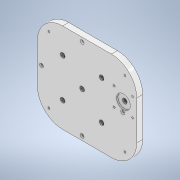
# Autodesk Inventor part: FourWireLitzBasePlate
Saved by Autodesk Inventor 2020.2 (Build 242310000, 310)
## iProperties
Created: 2020-03-15
Part Number: FourWireLitzBasePlate
Material: Generic
Document SubType Name: Modeling
Designer: elmar
Density: 1 g/cm^3
Appearance: White
Author: elmar
Autodesk Inventor part; units mm, degrees
ref_plane "YZ Plane" through (0, 0, 0) normal (1, 0, 0) x (0, 1, 0)
ref_plane "XZ Plane" through (0, 0, 0) normal (0, 1, 0) x (-1, 0, 0)
ref_plane "XY Plane" through (0, 0, 0) normal (0, 0, 1) x (1, 0, 0)
sketch "Sketch1" plane through (0, 0, 0) normal (0, 0, 1) x (1, 0, 0)
  line L0 (32.6, -32.6) -> (-32.6, -32.6)
  line L1 (-32.6, -32.6) -> (-32.6, 32.6)
  line L2 (-32.6, 32.6) -> (32.6, 32.6)
  line L3 (32.6, 32.6) -> (32.6, -32.6)
  line L4 (32.6, -32.6) -> (-32.6, 32.6) construction
  line L5 (-32.6, -32.6) -> (32.6, 32.6) construction
  line L6 (-67.9674, 0) -> (0, 67.9674)
  line L7 (0, 67.9674) -> (67.9674, 0)
  line L8 (67.9674, 0) -> (0, -67.9674)
  line L9 (0, -67.9674) -> (-67.9674, 0)
  line L10 (-108.2683, 0) -> (124.6095, 0) projected
  circle A0 centre (32.6, 32.6) radius 32.6
  circle A1 centre (69.1913, 15.9531) radius 7.6
  circle A2 centre (32.6, -32.6) radius 35
  circle A3 centre (69.1913, 15.9531) radius 10
  line L11 (53.6913, 31.4531) -> (84.6913, 31.4531)
  line L12 (84.6913, 31.4531) -> (84.6913, 0.4531)
  line L13 (84.6913, 0.4531) -> (53.6913, 0.4531)
  line L14 (53.6913, 0.4531) -> (53.6913, 31.4531)
  line L15 (90.3413, 37.1031) -> (90.3413, -5.1969)
  line L16 (90.3413, -5.1969) -> (48.0413, -5.1969)
  line L17 (48.0413, -5.1969) -> (48.0413, 37.1031)
  line L18 (48.0413, 37.1031) -> (90.3413, 37.1031)
  line L19 (-75, 75) -> (91.3413, 75)
  line L20 (91.3413, 75) -> (91.3413, -75)
  line L21 (91.3413, -75) -> (-75, -75)
  line L22 (-75, -75) -> (-75, 75)
  circle A4 centre (69.1913, 15.9531) radius 11.5
  circle A5 centre (67.9674, 0) radius 6
  point P0 (0, 0)
  point P1 (0, 0)
  point P2 (-75, 0)
  dimension "d0" = 65.2
  dimension "d1" = 67.9674
  dimension "d2" = 65.2
  dimension "d3" = 15.2
  dimension "d4" = 70
  dimension "d5" = 20
  dimension "d7" = 31
  dimension "d8" = 42.3
  dimension "d9" = 150
  dimension "d10" = 1
  dimension "d11" = 7.0326
  dimension "d12" = 7.0326
  dimension "d37" = 23
  dimension "d38" = 12
  dimension "d154" = 96.1204
  constraints: 44 end point, 8 coincident, 6 centre point, 4 parallel, 3 midpoint, 3 perpendicular, 2 horizontal, 2 point on line, 2 tangent, 2 vertical, 27 other
  measures "d0" distance of L1.end L2.end
  measures "d1" distance of point (0, 0) L6.start
  measures "d2" diameter of A0
  measures "d3" diameter of A1
  measures "d4" diameter of A2
  measures "d5" diameter of A3
  measures "d7" distance of L11.start L11.end
  measures "d8" distance of L17.end L15.start
  measures "d9" distance of L21.end L19.start
  measures "d10" distance between parallel lines of L20 L15
  measures "d11" distance from line of L19 L6.end
  measures "d12" distance from line of L22 L6.start
  measures "d37" diameter of A4
  measures "d38" diameter of A5
  measures "d154" distance of L8.end L6.start
extrude "Extrusion1" add sketch "Sketch1" along normal blind 10 contours L3 L10 A2 L17 L16 L8 L0 | L0 A2 L10 L3 | A2 L8 L9 L10 L1 L0 | L0 L1 L10 A2 | A0 A2 L3 | A0 A2 L10 | L10 A2 A0 | L3 A2 A0 | L10 L1 L2 A0 A2 | A2 L8 L16 A5 L15 L10 L20 L21 L22 L9 | L8 A2 | A2 A0 L2 L3 | L3 L2 A0 L7 L17 A2 | A2 A0 L17 L10 | L10 L17 A2 | L10 L6 L7 A0 L2 L1 | A2 L16 L8 | L17 A0 L14 L13 A5 L10 | L10 A5 L8 L16 A2 L17 | A2 L16 L17 | L17 L7 L14 A0 | L10 L22 L19 L20 L15 L18 A0 L7 L6 | L8 A5 L16 | A5 L13 L7 L10 | L10 L8 A5 | A0 L18 L17 L7 | L14 L7 A0 | A0 L7 A5 L13 L14 | L17 L18 A0 L11 L14 L7 | L8 L10 A5 L16 | L16 A5 | L7 L13 A5 L10 | A5 L7 L13 | L18 L15 L10 A5 L13 L12 L11 A0 | A0 A4 A5 L7 | L7 L14 L11 A0 A4 | A5 L10 L15 L16 | L7 A5 A4 L13 | A4 A0 A3 | A0 A3 A5 A4 | A5 A4 A0 L11 L12 L13 | A5 A4 | A3 A0 | A1 | A0 A3 | A4 A5 A3 A0
fillet "Fillet1" radius 42.4 4 edges at (-75, 75, 5) (91.3413, 75, 5) (91.3413, -75, 5) (-75, -75, 5)
hole "Hole1" at (84.6913, 31.4531, 0) at (53.6913, 31.4531, 0) at (53.6913, 0.4531, 0) at (84.6913, 0.4531, 0) direction (0, 0, 1) diameter 3.2 depth 10 tip angle 118 countersink diameter 6.5 countersink angle 90 clearance for "Flat Head Machine Screw" size "M3" standard "Ansi Metric M Profile"
sketch "Sketch2" plane through (0, 0, 10) normal (0, 0, 1) x (1, 0, 0)
  circle A0 centre (69.1913, 15.9531) radius 11.5 projected
  point P0 (0, 0)
  point P1 (0, 67.9674)
  point P2 (-67.9674, 0)
  point P3 (0, -67.9674)
  point P4 (67.9674, 0)
hole "Hole2" at (0, 67.9674, 10) at (67.9674, 0, 10) at (0, -67.9674, 10) at (-67.9674, 0, 10) direction (0, 0, -1) diameter 3.2 depth 10 tip angle 118 countersink diameter 6.5 countersink angle 90 clearance for "Flat Head Machine Screw" size "M3" standard "Ansi Metric M Profile"
hole "Hole3" at (32.6, 32.6, 0) at (69.1913, 15.9531, 0) at (32.6, -32.6, 0) at (-32.6, -32.6, 0) at (-32.6, 32.6, 0) at (0, 0, 0) direction (0, 0, 1) diameter 8 depth 10 tip angle 118
extrude "Extrusion2" cut sketch "Sketch2" against normal blind 2.2
sketch "Sketch3" plane through (0, 0, 0) normal (0, 0, -1) x (-1, 0, 0)
  line L0 (-71.8515, 55.5103) -> (55.5103, 55.5103)
  line L1 (55.5103, 55.5103) -> (55.5103, -55.5103)
  line L2 (55.5103, -55.5103) -> (-71.8515, -55.5103)
  line L3 (-71.8515, -55.5103) -> (-71.8515, 55.5103)
  line L4 (-71.8515, 55.5103) -> (-78.9226, 62.5813)
  arc A0 (-48.9413, 75) -> (-91.3413, 32.6) centre (-48.9413, 32.6) ccw projected
  line L5 (120.5621, 0) -> (-136.9034, 0) projected
  line L6 (55.5103, 55.5103) -> (62.5813, 62.5813)
  arc A1 (75, 32.6) -> (32.6, 75) centre (32.6, 32.6) ccw projected
  circle A2 centre (-69.1913, 15.9531) radius 4 projected
  line L7 (-90.3413, 37.1031) -> (-48.0413, 37.1031)
  line L8 (-48.0413, 37.1031) -> (-48.0413, -5.1969)
  line L9 (-48.0413, -5.1969) -> (-90.3413, -5.1969)
  line L10 (-90.3413, -5.1969) -> (-90.3413, 37.1031)
  point P0 (0, 0)
  point P1 (-71.8515, 0)
  dimension "d41" = 135
  dimension "d42" = 10
  dimension "d50" = 42.3
  constraints: 20 end point, 3 perpendicular, 2 horizontal, 2 parallel, 2 point on circle, 2 point on line, 1 coincident, 1 midpoint, 9 other
  measures "d41" angle of L0 L4
  measures "d42" distance of L0.start L4.end
  measures "d50" distance of L9.end L7.start
hole "Hole4" at (71.8515, 55.5103, 0) at (-55.5103, 55.5103, 0) at (-55.5103, -55.5103, 0) at (71.8515, -55.5103, 0) direction (0, 0, 1) diameter 3.2 depth 10 tip angle 118 countersink diameter 6.5 countersink angle 90 clearance for "Flat Head Machine Screw" size "M3" standard "Ansi Metric M Profile"
sketch "Sketch12" plane through (0, 0, 0) normal (0, 0, -1) x (-1, 0, 0)
  line L0 (-52.2872, 53.0579) -> (-50, 53.0579) construction
  line L1 (-50, 53.0579) -> (-50, 50) construction
  line L2 (-50, 50) -> (-52.2872, 50) construction
  line L3 (-52.2872, 50) -> (-52.2872, 53.0579) construction
  line L4 (50, 53.1122) -> (52.2872, 53.1122) construction
  line L5 (52.2872, 53.1122) -> (52.2872, 50) construction
  line L6 (52.2872, 50) -> (50, 50) construction
  line L7 (50, 50) -> (50, 53.1122) construction
  line L8 (50, -50) -> (52.2872, -50) construction
  line L9 (52.2872, -50) -> (52.2872, -53.1764) construction
  line L10 (52.2872, -53.1764) -> (50, -53.1764) construction
  line L11 (50, -53.1764) -> (50, -50) construction
  line L12 (-52.2872, -50) -> (-50, -50) construction
  line L13 (-50, -50) -> (-50, -53.048) construction
  line L14 (-50, -53.048) -> (-52.2872, -53.048) construction
  line L15 (-52.2872, -53.048) -> (-52.2872, -50) construction
  line L16 (-50, 50) -> (50, 50)
  line L17 (50, 50) -> (50, -50)
  line L18 (50, -50) -> (-50, -50)
  line L19 (-50, -50) -> (-50, 50)
  spline S0 degree 2 poles (-51.2424, 52.7047) (-51.3536, 52.7047) (-51.5734, 52.6503) (-51.6796, 52.6083) knots 0 0 0 1 2 2 2
  spline S1 degree 2 poles (-51.6796, 52.6083) (-51.7784, 52.5663) (-51.9241, 52.4774) (-51.981, 52.4379) knots 0 0 0 1 2 2 2
  line L20 (-51.981, 52.4379) -> (-52.0057, 52.4379)
  line L21 (-52.0057, 52.4379) -> (-52.0057, 52.8702)
  spline S2 degree 2 poles (-52.0057, 52.8702) (-51.8723, 52.9418) (-51.4153, 53.0579) (-51.2103, 53.0579) knots 0 0 0 1 2 2 2
  spline S3 degree 2 poles (-51.2103, 53.0579) (-51.0028, 53.0579) (-50.6941, 52.9739) (-50.5681, 52.885) knots 0 0 0 1 2 2 2
  spline S4 degree 2 poles (-50.5681, 52.885) (-50.4347, 52.7886) (-50.2964, 52.5095) (-50.2964, 52.3218) knots 0 0 0 1 2 2 2
  spline S5 degree 2 poles (-50.2964, 52.3218) (-50.2964, 52.0699) (-50.6274, 51.6895) (-50.8596, 51.6401) knots 0 0 0 1 2 2 2
  line L22 (-50.8596, 51.6401) -> (-50.8596, 51.6105)
  spline S6 degree 2 poles (-50.8596, 51.6105) (-50.7632, 51.5907) (-50.5434, 51.5018) (-50.4495, 51.4128) knots 0 0 0 1 2 2 2
  spline S7 degree 2 poles (-50.4495, 51.4128) (-50.3557, 51.3264) (-50.2371, 51.0498) (-50.2371, 50.8497) knots 0 0 0 1 2 2 2
  spline S8 degree 2 poles (-50.2371, 50.8497) (-50.2371, 50.6447) (-50.3779, 50.2964) (-50.5064, 50.163) knots 0 0 0 1 2 2 2
  spline S9 degree 2 poles (-50.5064, 50.163) (-50.6397, 50.0247) (-51.0176, 49.8814) (-51.2572, 49.8814) knots 0 0 0 1 2 2 2
  spline S10 degree 2 poles (-51.2572, 49.8814) (-51.4869, 49.8814) (-51.9365, 49.9926) (-52.0896, 50.0692) knots 0 0 0 1 2 2 2
  line L23 (-52.0896, 50.0692) -> (-52.0896, 50.5014)
  line L24 (-52.0896, 50.5014) -> (-52.06, 50.5014)
  spline S11 degree 2 poles (-52.06, 50.5014) (-51.9316, 50.4076) (-51.4968, 50.2347) (-51.2819, 50.2347) knots 0 0 0 1 2 2 2
  spline S12 degree 2 poles (-51.2819, 50.2347) (-51.156, 50.2347) (-50.904, 50.3137) (-50.82, 50.4051) knots 0 0 0 1 2 2 2
  spline S13 degree 2 poles (-50.82, 50.4051) (-50.7385, 50.4965) (-50.6521, 50.7138) (-50.6521, 50.8793) knots 0 0 0 1 2 2 2
  spline S14 degree 2 poles (-50.6521, 50.8793) (-50.6521, 51.0448) (-50.7484, 51.2597) (-50.8349, 51.3215) knots 0 0 0 1 2 2 2
  spline S15 degree 2 poles (-50.8349, 51.3215) (-50.9213, 51.3832) (-51.156, 51.4301) (-51.2943, 51.4301) knots 0 0 0 1 2 2 2
  line L25 (-51.2943, 51.4301) -> (-51.4672, 51.4301)
  line L26 (-51.4672, 51.4301) -> (-51.4672, 51.7685)
  line L27 (-51.4672, 51.7685) -> (-51.3313, 51.7685)
  spline S16 degree 2 poles (-51.3313, 51.7685) (-51.0572, 51.7685) (-50.7114, 52.0304) (-50.7114, 52.2798) knots 0 0 0 1 2 2 2
  spline S17 degree 2 poles (-50.7114, 52.2798) (-50.7114, 52.3959) (-50.8003, 52.5614) (-50.8719, 52.6108) knots 0 0 0 1 2 2 2
  spline S18 degree 2 poles (-50.8719, 52.6108) (-50.9485, 52.6627) (-51.1362, 52.7047) (-51.2424, 52.7047) knots 0 0 0 1 2 2 2
  line L28 (52.1835, 51.1115) -> (51.8204, 51.1115)
  line L29 (51.8204, 51.1115) -> (51.8204, 50.0642)
  line L30 (51.8204, 50.0642) -> (51.4277, 50.0642)
  line L31 (51.4277, 50.0642) -> (51.4277, 51.1115)
  line L32 (51.4277, 51.1115) -> (50.0815, 51.1115)
  line L33 (50.0815, 51.1115) -> (50.0815, 51.5413)
  line L34 (50.0815, 51.5413) -> (51.445, 53.1122)
  line L35 (51.445, 53.1122) -> (51.8204, 53.1122)
  line L36 (51.8204, 53.1122) -> (51.8204, 51.44)
  line L37 (51.8204, 51.44) -> (52.1835, 51.44)
  line L38 (52.1835, 51.44) -> (52.1835, 51.1115)
  line L39 (51.4277, 51.44) -> (51.4277, 52.6306)
  line L40 (51.4277, 52.6306) -> (50.4026, 51.44)
  line L41 (50.4026, 51.44) -> (51.4277, 51.44)
  line L42 (-50.1853, -53.1122) -> (-52.0649, -53.1122)
  line L43 (-52.0649, -53.1122) -> (-52.0649, -52.68)
  spline S19 degree 2 poles (-52.0649, -52.68) (-51.8624, -52.4898) (-51.5018, -52.1366) (-51.3289, -51.9464) knots 0 0 0 1 2 2 2
  spline S20 degree 2 poles (-51.3289, -51.9464) (-50.9806, -51.5635) (-50.7262, -51.1041) (-50.7262, -50.8596) knots 0 0 0 1 2 2 2
  spline S21 degree 2 poles (-50.7262, -50.8596) (-50.7262, -50.7311) (-50.8052, -50.5385) (-50.8769, -50.4767) knots 0 0 0 1 2 2 2
  spline S22 degree 2 poles (-50.8769, -50.4767) (-50.9485, -50.415) (-51.1362, -50.3532) (-51.2498, -50.3532) knots 0 0 0 1 2 2 2
  spline S23 degree 2 poles (-51.2498, -50.3532) (-51.3585, -50.3532) (-51.5808, -50.4076) (-51.6821, -50.4495) knots 0 0 0 1 2 2 2
  spline S24 degree 2 poles (-51.6821, -50.4495) (-51.7685, -50.4841) (-51.9291, -50.5829) (-51.9785, -50.6175) knots 0 0 0 1 2 2 2
  line L44 (-51.9785, -50.6175) -> (-52.0007, -50.6175)
  line L45 (-52.0007, -50.6175) -> (-52.0007, -50.1828)
  spline S25 degree 2 poles (-52.0007, -50.1828) (-51.8747, -50.121) (-51.4227, -50) (-51.2202, -50) knots 0 0 0 1 2 2 2
  spline S26 degree 2 poles (-51.2202, -50) (-50.7929, -50) (-50.3112, -50.452) (-50.3112, -50.8373) knots 0 0 0 1 2 2 2
  spline S27 degree 2 poles (-50.3112, -50.8373) (-50.3112, -51.0176) (-50.3952, -51.319) (-50.4693, -51.4474) knots 0 0 0 1 2 2 2
  spline S28 degree 2 poles (-50.4693, -51.4474) (-50.5434, -51.5808) (-50.7583, -51.8426) (-50.8769, -51.9686) knots 0 0 0 1 2 2 2
  spline S29 degree 2 poles (-50.8769, -51.9686) (-51.0695, -52.1786) (-51.5413, -52.6281) (-51.6821, -52.759) knots 0 0 0 1 2 2 2
  line L46 (-51.6821, -52.759) -> (-50.1853, -52.759)
  line L47 (-50.1853, -52.759) -> (-50.1853, -53.1122)
  line L48 (51.9488, -53.0579) -> (50.4619, -53.0579)
  line L49 (50.4619, -53.0579) -> (50.4619, -52.7467)
  line L50 (50.4619, -52.7467) -> (51.0152, -52.7467)
  line L51 (51.0152, -52.7467) -> (51.0152, -50.704)
  line L52 (51.0152, -50.704) -> (50.4619, -50.704)
  line L53 (50.4619, -50.704) -> (50.4619, -50.4248)
  spline S30 degree 2 poles (50.4619, -50.4248) (50.7756, -50.4248) (51.072, -50.247) (51.0917, -50) knots 0 0 0 1 2 2 2
  line L54 (51.0917, -50) -> (51.4079, -50)
  line L55 (51.4079, -50) -> (51.4079, -52.7467)
  line L56 (51.4079, -52.7467) -> (51.9488, -52.7467)
  line L57 (51.9488, -52.7467) -> (51.9488, -53.0579)
  point P0 (0, 0)
  point P1 (0, 0)
  dimension "d131" = 100
  constraints: 8 end point, 5 coincident, 1 vertical, 17 other
  measures "d131" distance of L16.start L16.end
emboss "Emboss1" sketch "Sketch12" operation cut depth 0.3 direction (0, 0, 1) contours S0 S1 L20 L21 S2 S3 S4 S5 L22 S6 S7 S8 S9 S10 L23 L24 S11 S12 S13 S14 S15 L25 L26 L27 S16 S17 S18 | L28 L29 L30 L31 L32 L33 L34 L35 L36 L37 L38 | L42 L43 S19 S20 S21 S22 S23 S24 L44 L45 S25 S26 S27 S28 S29 L46 L47 | L48 L49 L50 L51 L52 L53 S30 L54 L55 L56 L57
thread "Thread6" size "M8x1.25" class "6H" standard "ANSI Metric M Profile" full length
thread "Thread7" size "M8x1.25" class "6H" standard "ANSI Metric M Profile" full length
thread "Thread8" size "M8x1.25" class "6H" standard "ANSI Metric M Profile" full length
thread "Thread9" size "M8x1.25" class "6H" standard "ANSI Metric M Profile" full length
thread "Thread10" size "M8x1.25" class "6H" standard "ANSI Metric M Profile" full length
sketch "Sketch48" plane through (32.6, 32.6, 10) normal (-1, 0, 0) x (0, 1, 0)
  line L0 (4, 0) -> (4, 10)
  line L1 (4, 10) -> (3.0732, 10)
  line L2 (3.0732, 10) -> (3.0732, 0)
  line L3 (3.0732, 0) -> (4, 0)
  line L4 (0, -2) -> (0, 12) projected
  constraints: 8 end point
revolve "Revolution21" add sketch "Sketch48" angle 360 about axis through (32.6, 32.6, 10) along (0, 0, -1) separate body
sketch "Sketch47" plane through (32.6, 36.6, 10) normal (1, 0, 0) x (0, 0, -1)
  line L0 (-0.7293, -0.0634) -> (-0.6251, -0.0634) construction
  line L1 (0.1041, -0.8638) -> (-0.0001, -1.0639) construction
  line L2 (-1.2501, -1.0639) -> (-1.3543, -0.8638) construction
  line L3 (-0.5209, -0.0634) -> (-0.6251, 0.1367) construction
  line L4 (-0.6251, 0.1367) -> (-0.7293, -0.0634) construction
  line L5 (-1.2501, -1.0639) -> (-1.1459, -0.8638) construction
  line L6 (-0.5209, -0.0634) -> (-0.1043, -0.8638)
  line L7 (-1.3543, -0.8638) -> (-1.1459, -0.8638) construction
  arc A0 (-1.3543, -0.8638) -> (-1.2501, -0.927) centre (-1.2501, -0.8096) ccw construction
  line L8 (0.1041, -0.8638) -> (-0.1043, -0.8638) construction
  line L9 (-1.2501, -1.0639) -> (-1.2501, -0.8638) construction
  line L10 (-0.0001, -1.0639) -> (-0.0001, -0.8638) construction
  line L11 (-0.6251, 0.1367) -> (-0.6251, -0.0002) construction
  line L12 (-1.2501, -0.927) -> (-0.0001, -0.927)
  arc A1 (-1.2501, -0.927) -> (-1.1459, -0.8638) centre (-1.2501, -0.8096) ccw
  line L13 (-0.1043, -0.8638) -> (-0.0001, -1.0639) construction
  line L14 (-1.1459, -0.8638) -> (-0.7293, -0.0634)
  line L15 (-0.0001, -0.0002) -> (-0.0001, 0.0177)
  line L16 (-0.0001, 0.0177) -> (-0.0001, -0.0002)
  line L17 (-0.0001, -0.0002) -> (0.0334, -0.0002)
  arc A2 (-0.1043, -0.8638) -> (-0.0001, -0.927) centre (-0.0001, -0.8096) ccw
  arc A3 (-0.0001, -0.927) -> (0.1041, -0.8638) centre (-0.0001, -0.8096) ccw construction
  arc A4 (-0.6251, -0.0002) -> (-0.7293, -0.0634) centre (-0.6251, -0.1176) ccw
  arc A5 (-0.5209, -0.0634) -> (-0.6251, -0.0002) centre (-0.6251, -0.1176) ccw
  line L18 (-0.6251, -0.0002) -> (-0.6251, -0.0634) construction
  line L19 (-0.6251, -0.0634) -> (-0.5209, -0.0634) construction
  dimension "d459" = 55
  dimension "d460" = 0.2001
  dimension "d461" = 0.2001
  dimension "Sketch47_ThreadOffset" = 0
  dimension "Sketch47_MajorRadius" = 0.9268
  dimension "d464" = 1.25
  dimension "Sketch47_MinorRadius" = 0
  constraints: 40 end point, 12 point on circle, 10 parallel, 8 tangent, 6 centre point, 6 collinear, 2 midpoint, 2 point on line, 1 horizontal, 1 perpendicular, 3 other
  measures "d459" angle of L6 L14
  measures "d460" distance of L3.end L0.end
  measures "d461" distance of L1.end L10.end
  measures "Sketch47_ThreadOffset" distance between parallel lines of L15 L10
  measures "Sketch47_MajorRadius" distance from line of L12 L15.start
  measures "d464" distance from line of L1.end L9
  measures "Sketch47_MinorRadius" distance edge to line of A5 L17
coil "Coil21" sketch "Sketch47" operation cut axis through (32.6, 32.6, 10) along (0, 0, -1) pitch 1.2513 turns 9.99001 hand right bodies 2
sketch "Sketch50" plane through (-32.6, 32.6, 10) normal (-1, 0, 0) x (0, 1, 0)
  line L0 (4, 0) -> (4, 10)
  line L1 (4, 10) -> (3.0732, 10)
  line L2 (3.0732, 10) -> (3.0732, 0)
  line L3 (3.0732, 0) -> (4, 0)
  line L4 (0, -2) -> (0, 12) projected
  constraints: 8 end point
revolve "Revolution22" add sketch "Sketch50" angle 360 about axis through (-32.6, 32.6, 10) along (0, 0, -1) separate body
sketch "Sketch49" plane through (-32.6, 36.6, 10) normal (1, 0, 0) x (0, 0, -1)
  line L0 (-0.7293, -0.0634) -> (-0.6251, -0.0634) construction
  line L1 (0.1041, -0.8638) -> (-0.0001, -1.0639) construction
  line L2 (-1.2501, -1.0639) -> (-1.3543, -0.8638) construction
  line L3 (-0.5209, -0.0634) -> (-0.6251, 0.1367) construction
  line L4 (-0.6251, 0.1367) -> (-0.7293, -0.0634) construction
  line L5 (-1.2501, -1.0639) -> (-1.1459, -0.8638) construction
  line L6 (-0.5209, -0.0634) -> (-0.1043, -0.8638)
  line L7 (-1.3543, -0.8638) -> (-1.1459, -0.8638) construction
  arc A0 (-1.3543, -0.8638) -> (-1.2501, -0.927) centre (-1.2501, -0.8096) ccw construction
  line L8 (0.1041, -0.8638) -> (-0.1043, -0.8638) construction
  line L9 (-1.2501, -1.0639) -> (-1.2501, -0.8638) construction
  line L10 (-0.0001, -1.0639) -> (-0.0001, -0.8638) construction
  line L11 (-0.6251, 0.1367) -> (-0.6251, -0.0002) construction
  line L12 (-1.2501, -0.927) -> (-0.0001, -0.927)
  arc A1 (-1.2501, -0.927) -> (-1.1459, -0.8638) centre (-1.2501, -0.8096) ccw
  line L13 (-0.1043, -0.8638) -> (-0.0001, -1.0639) construction
  line L14 (-1.1459, -0.8638) -> (-0.7293, -0.0634)
  line L15 (-0.0001, -0.0002) -> (-0.0001, 0.0177)
  line L16 (-0.0001, 0.0177) -> (-0.0001, -0.0002)
  line L17 (-0.0001, -0.0002) -> (0.0334, -0.0002)
  arc A2 (-0.1043, -0.8638) -> (-0.0001, -0.927) centre (-0.0001, -0.8096) ccw
  arc A3 (-0.0001, -0.927) -> (0.1041, -0.8638) centre (-0.0001, -0.8096) ccw construction
  arc A4 (-0.6251, -0.0002) -> (-0.7293, -0.0634) centre (-0.6251, -0.1176) ccw
  arc A5 (-0.5209, -0.0634) -> (-0.6251, -0.0002) centre (-0.6251, -0.1176) ccw
  line L18 (-0.6251, -0.0002) -> (-0.6251, -0.0634) construction
  line L19 (-0.6251, -0.0634) -> (-0.5209, -0.0634) construction
  dimension "d477" = 55
  dimension "d478" = 0.2001
  dimension "d479" = 0.2001
  dimension "Sketch49_ThreadOffset" = 0
  dimension "Sketch49_MajorRadius" = 0.9268
  dimension "d482" = 1.25
  dimension "Sketch49_MinorRadius" = 0
  constraints: 40 end point, 12 point on circle, 10 parallel, 8 tangent, 6 centre point, 6 collinear, 2 midpoint, 2 point on line, 1 horizontal, 1 perpendicular, 3 other
  measures "d477" angle of L6 L14
  measures "d478" distance of L3.end L0.end
  measures "d479" distance of L1.end L10.end
  measures "Sketch49_ThreadOffset" distance between parallel lines of L15 L10
  measures "Sketch49_MajorRadius" distance from line of L12 L15.start
  measures "d482" distance from line of L1.end L9
  measures "Sketch49_MinorRadius" distance edge to line of A5 L17
coil "Coil22" sketch "Sketch49" operation cut axis through (-32.6, 32.6, 10) along (0, 0, -1) pitch 1.2513 turns 9.99001 hand right bodies 3
sketch "Sketch52" plane through (0, 0, 10) normal (-1, 0, 0) x (0, 1, 0)
  line L0 (4, 0) -> (4, 10)
  line L1 (4, 10) -> (3.0732, 10)
  line L2 (3.0732, 10) -> (3.0732, 0)
  line L3 (3.0732, 0) -> (4, 0)
  line L4 (0, -2) -> (0, 12) projected
  constraints: 8 end point
revolve "Revolution23" add sketch "Sketch52" angle 360 about axis through (0, 0, 10) along (0, 0, -1) separate body
sketch "Sketch51" plane through (0, 4, 10) normal (1, 0, 0) x (0, 0, -1)
  line L0 (-0.7293, -0.0634) -> (-0.6251, -0.0634) construction
  line L1 (0.1041, -0.8638) -> (-0.0001, -1.0639) construction
  line L2 (-1.2501, -1.0639) -> (-1.3543, -0.8638) construction
  line L3 (-0.5209, -0.0634) -> (-0.6251, 0.1367) construction
  line L4 (-0.6251, 0.1367) -> (-0.7293, -0.0634) construction
  line L5 (-1.2501, -1.0639) -> (-1.1459, -0.8638) construction
  line L6 (-0.5209, -0.0634) -> (-0.1043, -0.8638)
  line L7 (-1.3543, -0.8638) -> (-1.1459, -0.8638) construction
  arc A0 (-1.3543, -0.8638) -> (-1.2501, -0.927) centre (-1.2501, -0.8096) ccw construction
  line L8 (0.1041, -0.8638) -> (-0.1043, -0.8638) construction
  line L9 (-1.2501, -1.0639) -> (-1.2501, -0.8638) construction
  line L10 (-0.0001, -1.0639) -> (-0.0001, -0.8638) construction
  line L11 (-0.6251, 0.1367) -> (-0.6251, -0.0002) construction
  line L12 (-1.2501, -0.927) -> (-0.0001, -0.927)
  arc A1 (-1.2501, -0.927) -> (-1.1459, -0.8638) centre (-1.2501, -0.8096) ccw
  line L13 (-0.1043, -0.8638) -> (-0.0001, -1.0639) construction
  line L14 (-1.1459, -0.8638) -> (-0.7293, -0.0634)
  line L15 (-0.0001, -0.0002) -> (-0.0001, 0.0177)
  line L16 (-0.0001, 0.0177) -> (-0.0001, -0.0002)
  line L17 (-0.0001, -0.0002) -> (0.0334, -0.0002)
  arc A2 (-0.1043, -0.8638) -> (-0.0001, -0.927) centre (-0.0001, -0.8096) ccw
  arc A3 (-0.0001, -0.927) -> (0.1041, -0.8638) centre (-0.0001, -0.8096) ccw construction
  arc A4 (-0.6251, -0.0002) -> (-0.7293, -0.0634) centre (-0.6251, -0.1176) ccw
  arc A5 (-0.5209, -0.0634) -> (-0.6251, -0.0002) centre (-0.6251, -0.1176) ccw
  line L18 (-0.6251, -0.0002) -> (-0.6251, -0.0634) construction
  line L19 (-0.6251, -0.0634) -> (-0.5209, -0.0634) construction
  dimension "d495" = 55
  dimension "d496" = 0.2001
  dimension "d497" = 0.2001
  dimension "Sketch51_ThreadOffset" = 0
  dimension "Sketch51_MajorRadius" = 0.9268
  dimension "d500" = 1.25
  dimension "Sketch51_MinorRadius" = 0
  constraints: 40 end point, 12 point on circle, 10 parallel, 8 tangent, 6 centre point, 6 collinear, 2 midpoint, 2 point on line, 1 horizontal, 1 perpendicular, 3 other
  measures "d495" angle of L6 L14
  measures "d496" distance of L3.end L0.end
  measures "d497" distance of L1.end L10.end
  measures "Sketch51_ThreadOffset" distance between parallel lines of L15 L10
  measures "Sketch51_MajorRadius" distance from line of L12 L15.start
  measures "d500" distance from line of L1.end L9
  measures "Sketch51_MinorRadius" distance edge to line of A5 L17
coil "Coil23" sketch "Sketch51" operation cut axis through (0, 0, 10) along (0, 0, -1) pitch 1.2513 turns 9.99001 hand right bodies 4
sketch "Sketch54" plane through (32.6, -32.6, 10) normal (-1, 0, 0) x (0, 1, 0)
  line L0 (4, 0) -> (4, 10)
  line L1 (4, 10) -> (3.0732, 10)
  line L2 (3.0732, 10) -> (3.0732, 0)
  line L3 (3.0732, 0) -> (4, 0)
  line L4 (0, -2) -> (0, 12) projected
  constraints: 8 end point
revolve "Revolution24" add sketch "Sketch54" angle 360 about axis through (32.6, -32.6, 10) along (0, 0, -1) separate body
sketch "Sketch53" plane through (32.6, -28.6, 10) normal (1, 0, 0) x (0, 0, -1)
  line L0 (-0.7293, -0.0634) -> (-0.6251, -0.0634) construction
  line L1 (0.1041, -0.8638) -> (-0.0001, -1.0639) construction
  line L2 (-1.2501, -1.0639) -> (-1.3543, -0.8638) construction
  line L3 (-0.5209, -0.0634) -> (-0.6251, 0.1367) construction
  line L4 (-0.6251, 0.1367) -> (-0.7293, -0.0634) construction
  line L5 (-1.2501, -1.0639) -> (-1.1459, -0.8638) construction
  line L6 (-0.5209, -0.0634) -> (-0.1043, -0.8638)
  line L7 (-1.3543, -0.8638) -> (-1.1459, -0.8638) construction
  arc A0 (-1.3543, -0.8638) -> (-1.2501, -0.927) centre (-1.2501, -0.8096) ccw construction
  line L8 (0.1041, -0.8638) -> (-0.1043, -0.8638) construction
  line L9 (-1.2501, -1.0639) -> (-1.2501, -0.8638) construction
  line L10 (-0.0001, -1.0639) -> (-0.0001, -0.8638) construction
  line L11 (-0.6251, 0.1367) -> (-0.6251, -0.0002) construction
  line L12 (-1.2501, -0.927) -> (-0.0001, -0.927)
  arc A1 (-1.2501, -0.927) -> (-1.1459, -0.8638) centre (-1.2501, -0.8096) ccw
  line L13 (-0.1043, -0.8638) -> (-0.0001, -1.0639) construction
  line L14 (-1.1459, -0.8638) -> (-0.7293, -0.0634)
  line L15 (-0.0001, -0.0002) -> (-0.0001, 0.0177)
  line L16 (-0.0001, 0.0177) -> (-0.0001, -0.0002)
  line L17 (-0.0001, -0.0002) -> (0.0334, -0.0002)
  arc A2 (-0.1043, -0.8638) -> (-0.0001, -0.927) centre (-0.0001, -0.8096) ccw
  arc A3 (-0.0001, -0.927) -> (0.1041, -0.8638) centre (-0.0001, -0.8096) ccw construction
  arc A4 (-0.6251, -0.0002) -> (-0.7293, -0.0634) centre (-0.6251, -0.1176) ccw
  arc A5 (-0.5209, -0.0634) -> (-0.6251, -0.0002) centre (-0.6251, -0.1176) ccw
  line L18 (-0.6251, -0.0002) -> (-0.6251, -0.0634) construction
  line L19 (-0.6251, -0.0634) -> (-0.5209, -0.0634) construction
  dimension "d513" = 55
  dimension "d514" = 0.2001
  dimension "d515" = 0.2001
  dimension "Sketch53_ThreadOffset" = 0
  dimension "Sketch53_MajorRadius" = 0.9268
  dimension "d518" = 1.25
  dimension "Sketch53_MinorRadius" = 0
  constraints: 40 end point, 12 point on circle, 10 parallel, 8 tangent, 6 centre point, 6 collinear, 2 midpoint, 2 point on line, 1 horizontal, 1 perpendicular, 3 other
  measures "d513" angle of L6 L14
  measures "d514" distance of L3.end L0.end
  measures "d515" distance of L1.end L10.end
  measures "Sketch53_ThreadOffset" distance between parallel lines of L15 L10
  measures "Sketch53_MajorRadius" distance from line of L12 L15.start
  measures "d518" distance from line of L1.end L9
  measures "Sketch53_MinorRadius" distance edge to line of A5 L17
coil "Coil24" sketch "Sketch53" operation cut axis through (32.6, -32.6, 10) along (0, 0, -1) pitch 1.2513 turns 9.99001 hand right bodies 5
sketch "Sketch56" plane through (-32.6, -32.6, 10) normal (-1, 0, 0) x (0, 1, 0)
  line L0 (4, 0) -> (4, 10)
  line L1 (4, 10) -> (3.0732, 10)
  line L2 (3.0732, 10) -> (3.0732, 0)
  line L3 (3.0732, 0) -> (4, 0)
  line L4 (0, -2) -> (0, 12) projected
  constraints: 8 end point
revolve "Revolution25" add sketch "Sketch56" angle 360 about axis through (-32.6, -32.6, 10) along (0, 0, -1) separate body
sketch "Sketch55" plane through (-32.6, -28.6, 10) normal (1, 0, 0) x (0, 0, -1)
  line L0 (-0.7293, -0.0634) -> (-0.6251, -0.0634) construction
  line L1 (0.1041, -0.8638) -> (-0.0001, -1.0639) construction
  line L2 (-1.2501, -1.0639) -> (-1.3543, -0.8638) construction
  line L3 (-0.5209, -0.0634) -> (-0.6251, 0.1367) construction
  line L4 (-0.6251, 0.1367) -> (-0.7293, -0.0634) construction
  line L5 (-1.2501, -1.0639) -> (-1.1459, -0.8638) construction
  line L6 (-0.5209, -0.0634) -> (-0.1043, -0.8638)
  line L7 (-1.3543, -0.8638) -> (-1.1459, -0.8638) construction
  arc A0 (-1.3543, -0.8638) -> (-1.2501, -0.927) centre (-1.2501, -0.8096) ccw construction
  line L8 (0.1041, -0.8638) -> (-0.1043, -0.8638) construction
  line L9 (-1.2501, -1.0639) -> (-1.2501, -0.8638) construction
  line L10 (-0.0001, -1.0639) -> (-0.0001, -0.8638) construction
  line L11 (-0.6251, 0.1367) -> (-0.6251, -0.0002) construction
  line L12 (-1.2501, -0.927) -> (-0.0001, -0.927)
  arc A1 (-1.2501, -0.927) -> (-1.1459, -0.8638) centre (-1.2501, -0.8096) ccw
  line L13 (-0.1043, -0.8638) -> (-0.0001, -1.0639) construction
  line L14 (-1.1459, -0.8638) -> (-0.7293, -0.0634)
  line L15 (-0.0001, -0.0002) -> (-0.0001, 0.0177)
  line L16 (-0.0001, 0.0177) -> (-0.0001, -0.0002)
  line L17 (-0.0001, -0.0002) -> (0.0334, -0.0002)
  arc A2 (-0.1043, -0.8638) -> (-0.0001, -0.927) centre (-0.0001, -0.8096) ccw
  arc A3 (-0.0001, -0.927) -> (0.1041, -0.8638) centre (-0.0001, -0.8096) ccw construction
  arc A4 (-0.6251, -0.0002) -> (-0.7293, -0.0634) centre (-0.6251, -0.1176) ccw
  arc A5 (-0.5209, -0.0634) -> (-0.6251, -0.0002) centre (-0.6251, -0.1176) ccw
  line L18 (-0.6251, -0.0002) -> (-0.6251, -0.0634) construction
  line L19 (-0.6251, -0.0634) -> (-0.5209, -0.0634) construction
  dimension "d531" = 55
  dimension "d532" = 0.2001
  dimension "d533" = 0.2001
  dimension "Sketch55_ThreadOffset" = 0
  dimension "Sketch55_MajorRadius" = 0.9268
  dimension "d536" = 1.25
  dimension "Sketch55_MinorRadius" = 0
  constraints: 40 end point, 12 point on circle, 10 parallel, 8 tangent, 6 centre point, 6 collinear, 2 midpoint, 2 point on line, 1 horizontal, 1 perpendicular, 3 other
  measures "d531" angle of L6 L14
  measures "d532" distance of L3.end L0.end
  measures "d533" distance of L1.end L10.end
  measures "Sketch55_ThreadOffset" distance between parallel lines of L15 L10
  measures "Sketch55_MajorRadius" distance from line of L12 L15.start
  measures "d536" distance from line of L1.end L9
  measures "Sketch55_MinorRadius" distance edge to line of A5 L17
coil "Coil25" sketch "Sketch55" operation cut axis through (-32.6, -32.6, 10) along (0, 0, -1) pitch 1.2513 turns 9.99001 hand right bodies 6
equation "\"d0\" = ReferenceDiameter + GearClearance"
equation "\"d2\" = ReferenceDiameter + GearClearance"
equation "\"d4\" = TipDiameter_1"
equation "\"d5\" = TipDiameter"
equation "\"d9\" = SideLength"
equation "\"d12\" = d11"
equation "\"d15\" = CornerRadius"
equation "\"d1\" = SupportHoleDistance"
equation "\"d459\" = d466"
equation "\"d460\" = 0.160083 * Sketch47_Pitch"
equation "\"d461\" = 0.160083 * Sketch47_Pitch"
equation "\"d464\" = Sketch47_Pitch"
equation "\"d477\" = d484"
equation "\"d478\" = 0.160083 * Sketch49_Pitch"
equation "\"d479\" = 0.160083 * Sketch49_Pitch"
equation "\"d482\" = Sketch49_Pitch"
equation "\"d495\" = d502"
equation "\"d496\" = 0.160083 * Sketch51_Pitch"
equation "\"d497\" = 0.160083 * Sketch51_Pitch"
equation "\"d500\" = Sketch51_Pitch"
equation "\"d513\" = d520"
equation "\"d514\" = 0.160083 * Sketch53_Pitch"
equation "\"d515\" = 0.160083 * Sketch53_Pitch"
equation "\"d518\" = Sketch53_Pitch"
equation "\"d531\" = d538"
equation "\"d532\" = 0.160083 * Sketch55_Pitch"
equation "\"d533\" = 0.160083 * Sketch55_Pitch"
equation "\"d536\" = Sketch55_Pitch"
equation "\"d66\" = 55deg"
equation "\"Sketch4_Pitch\" = 1.25"
equation "\"d84\" = 55deg"
equation "\"Sketch6_Pitch\" = 1.25"
equation "\"d102\" = 55deg"
equation "\"Sketch8_Pitch\" = 1.25"
equation "\"d120\" = 55deg"
equation "\"Sketch10_Pitch\" = 1.25"
equation "\"d143\" = 55deg"
equation "\"Sketch13_Pitch\" = 1.25"
equation "\"GearClearance\" = 0.2"
equation "\"d162\" = 55deg"
equation "\"Sketch15_Pitch\" = 1.25"
equation "\"d180\" = 55deg"
equation "\"Sketch17_Pitch\" = 1.25"
equation "\"d198\" = 55deg"
equation "\"Sketch19_Pitch\" = 1.25"
equation "\"d216\" = 55deg"
equation "\"Sketch21_Pitch\" = 1.25"
equation "\"d234\" = 55deg"
equation "\"Sketch23_Pitch\" = 1.25"
equation "\"d262\" = 55deg"
equation "\"Sketch25_Pitch\" = 1.25"
equation "\"d280\" = 55deg"
equation "\"Sketch27_Pitch\" = 1.25"
equation "\"d298\" = 55deg"
equation "\"Sketch29_Pitch\" = 1.25"
equation "\"d316\" = 55deg"
equation "\"Sketch31_Pitch\" = 1.25"
equation "\"d334\" = 55deg"
equation "\"Sketch33_Pitch\" = 1.25"
equation "\"d376\" = 55deg"
equation "\"Sketch37_Pitch\" = 1.25"
equation "\"d394\" = 55deg"
equation "\"Sketch39_Pitch\" = 1.25"
equation "\"d412\" = 55deg"
equation "\"Sketch41_Pitch\" = 1.25"
equation "\"d430\" = 55deg"
equation "\"Sketch43_Pitch\" = 1.25"
equation "\"d448\" = 55deg"
equation "\"Sketch45_Pitch\" = 1.25"
equation "\"d466\" = 55deg"
equation "\"Sketch47_Pitch\" = 1.25"
equation "\"d484\" = 55deg"
equation "\"Sketch49_Pitch\" = 1.25"
equation "\"d502\" = 55deg"
equation "\"Sketch51_Pitch\" = 1.25"
equation "\"d520\" = 55deg"
equation "\"Sketch53_Pitch\" = 1.25"
equation "\"d538\" = 55deg"
equation "\"Sketch55_Pitch\" = 1.25"
equation "\"ReferenceDiameter\" = 65"
equation "\"TipDiameter_1\" = 70"
equation "\"TipDiameter\" = 20"
equation "\"SideLength\" = 150"
equation "\"CornerRadius\" = 42.4"
equation "\"SupportHoleDistance\" = 67.967358"
body "Solid1"
body "Solid22"
body "Solid23"
body "Solid24"
body "Solid25"
body "Solid26"
